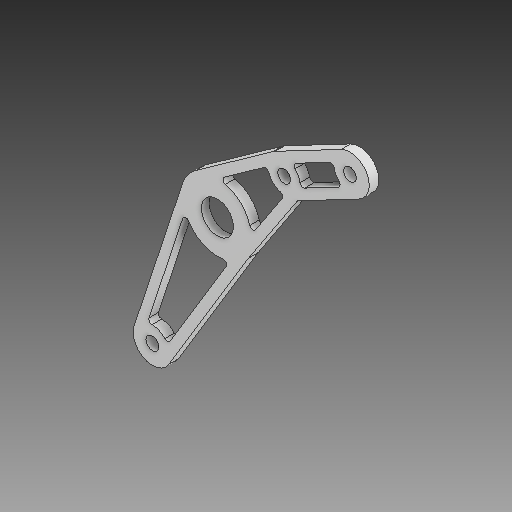
# Autodesk Inventor part: アーム軸抑え3
Saved by Autodesk Inventor 2020 (Build 240168000, 168)
## iProperties
Created: 2019-09-05
Part Number: アーム軸抑え3
Material: アルミニウム 2014-T4
Document SubType Name: Modeling
Designer: 雪村
Density: 2.8 g/cm^3
Appearance: サテン
Mass: 8.59692 g
Surface Area: 35.8283 cm^2
Volume: 3.07033 cm^3
Description: アルミ2000 3t
Author: 雪村
Autodesk Inventor part; units mm, degrees
ref_plane "YZ Plane" through (0, 0, 0) normal (1, 0, 0) x (0, 1, 0)
ref_plane "XZ Plane" through (0, 0, 0) normal (0, 1, 0) x (-1, 0, 0)
ref_plane "XY Plane" through (0, 0, 0) normal (0, 0, 1) x (1, 0, 0)
sketch "スケッチ1" plane through (0, 0, 0) normal (0, 0, 1) x (1, 0, 0)
  circle A0 centre (-73.413, 50.8387) radius 2
  circle A1 centre (-11.7367, 127.3646) radius 2
  circle A2 centre (-32.2967, 116.5802) radius 2
  circle A3 centre (-53.1365, 95) radius 5.025
  circle A4 centre (-11.7367, 127.3646) radius 6
  circle A5 centre (-32.2967, 116.5802) radius 6
  circle A6 centre (-53.1365, 95) radius 11.5
  circle A7 centre (-73.413, 50.8387) radius 6
  line L0 (-79.114, 52.7091) -> (-64.0635, 98.5848)
  line L1 (-59.8041, 104.3698) -> (-35.7755, 121.4688)
  line L2 (-35.0838, 121.8936) -> (-14.5238, 132.678)
  line L3 (-29.5097, 111.2668) -> (-8.9496, 122.0512)
  line L4 (-27.2897, 113.2742) -> (-43.5397, 88.6634)
  line L5 (-43.2957, 89.0494) -> (-68.2786, 47.734)
  circle A8 centre (-53.1365, 95) radius 7.5
  point P0 (0, 0)
  point P1 (-43.4139, 88.854)
  point P2 (-28.1412, 111.9846)
  dimension "d0" = 4
  dimension "d1" = 4
  dimension "d2" = 4
  dimension "d3" = 10.05
  dimension "d4" = 4
  dimension "d5" = 4
  dimension "d7" = 4
  dimension "d15" = 15
  dimension "d16" = 4
  constraints: 12 end point, 12 point on circle, 12 tangent, 9 centre point, 2 coincident, 4 other
  measures "d0" diameter of A0
  measures "d1" diameter of A1
  measures "d2" diameter of A2
  measures "d3" diameter of A3
  measures "d4" radial gap between concentric circles of A1 A4
  measures "d5" radial gap between concentric circles of A2 A5
  measures "d7" radial gap between concentric circles of A0 A7
  measures "d15" diameter of A8
  measures "d16" radial gap between concentric circles of A6 A8
extrude "押し出し1" add sketch "スケッチ1" along normal blind 3 contours A4 | A4 L3 L4 A5 L2 | A5 | L4 L5 A6 L1 A5 L3 | L3 A5 L4 | L5 A7 L0 A6 L4 | L4 A6 L5 | A6 | A7 | A8
sketch "スケッチ2" plane through (0, 0, 0) normal (0, 0, -1) x (-1, 0, 0)
  circle A0 centre (53.1365, 95) radius 5.025 projected
  circle A1 centre (53.1365, 95) radius 7.5
  point P0 (0, 0)
  dimension "d12" = 15
  constraints: 1 centre point, 1 coincident
  measures "d12" diameter of A1
extrude "押し出し2" cut sketch "スケッチ2" against normal blind 0.5
shell "シェル2" thickness 3 removed faces 2 at (-67.6516, 80.9362, 0) at (-66.6917, 80.9872, 3)
fillet "フィレット2" radius 1 19 edges at (-43.4139, 88.854, 1.5) (-28.1412, 111.9846, 1.5) (-75.0166, 55.5746, 1.5) (-63.1345, 91.7924, 1.75) (-63.1345, 91.7924, 0.25) (-68.776, 52.7092, 1.5) (-49.0526, 85.3267, 0.25) (-49.0526, 85.3267, 1.75) (-45.6365, 95, 0.5) (-53.0422, 105.4996, 0.25) (-53.0422, 105.4996, 1.75) (-37.2952, 116.7053, 1.5) (-42.6466, 95.4607, 0.25) (-31.9972, 111.5892, 1.5) (-42.6466, 95.4607, 1.75) (-30.148, 121.0949, 1.5) (-16.6725, 128.1633, 1.5) (-27.3609, 115.7815, 1.5) (-13.8854, 122.8499, 1.5)
sketch "スケッチ3" plane through (0, 0, 0) normal (0, 0, -1) x (-1, 0, 0)
  circle A0 centre (53.1365, 95) radius 5.025 projected
  circle A1 centre (53.1365, 95) radius 7.5
  point P0 (0, 0)
  dimension "d19" = 15
  constraints: 1 centre point, 1 coincident
  measures "d19" diameter of A1
extrude "押し出し3" cut sketch "スケッチ3" against normal blind 0.5 contours A0 | A1
